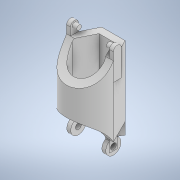
# Autodesk Inventor part: 검지_손가락_아래
Saved by Autodesk Inventor 2022 (Build 260153000, 153)
## iProperties
Created: 2023-11-18
Part Number: 검지_손가락_아래
Material: 일반
Document SubType Name: Modeling
Designer: USER
Density: 1 g/cm^3
Appearance: 기본값
Author: USER
Autodesk Inventor part; units mm, degrees
ref_plane "YZ Plane" through (0, 0, 0) normal (1, 0, 0) x (0, 1, 0)
ref_plane "XZ Plane" through (0, 0, 0) normal (0, 1, 0) x (-1, 0, 0)
ref_plane "XY Plane" through (0, 0, 0) normal (0, 0, 1) x (1, 0, 0)
sketch "스케치1" plane through (0, 0, 0) normal (0, 1, 0) x (-1, 0, 0)
  line L0 (0, 0) -> (0, -20)
  line L1 (0, -10) -> (-10, -10)
  line L2 (0, -20) -> (-5, -20)
  line L3 (-5, -20) -> (-10, -10)
  arc A0 (0, 0) -> (-10, -10) centre (0, -10) ccw
  line L4 (0, -20) -> (5, -20)
  line L5 (5, -20) -> (10, -10)
  arc A1 (10, -10) -> (0, 0) centre (0, -10) ccw
  dimension "d0" = 20
  dimension "d1" = 10
  dimension "d2" = 5
  constraints: 12 end point, 4 point on circle, 2 centre point, 2 horizontal, 2 symmetric about line, 1 coincident, 1 midpoint, 1 point on line, 1 vertical, 1 other
  measures "d0" distance of L0.start L0.end
  measures "d1" distance of L1.end L1.start
  measures "d2" distance of L0.end L2.end
extrude "돌출1" add sketch "스케치1" along normal blind 30
sketch "스케치7" plane through (0, 0, 0) normal (1, 0, 0) x (0, 1, 0)
  line L0 (30, -10) -> (30, 0) projected
  line L1 (30, 0) -> (21, 0)
  line L2 (0, 0) -> (30, 0) projected
  line L3 (21, 0) -> (25.4109, -9.3555) construction
  line L4 (25.4109, -9.3555) -> (35.2847, -12.2144) construction
  spline S0 degree 2 poles (21, 0) (25.4109, -9.3555) (35.2847, -12.2144) knots 1 1 1 2 2 2
  line L5 (35.2847, -12.2144) -> (35.2847, 0)
  line L6 (35.2847, 0) -> (21, 0)
  line L7 (15, 0) -> (15, 13.9402)
  line L8 (-5.2847, 0) -> (9, 0)
  line L9 (0, -10) -> (30, -10) projected
  line L10 (9, 0) -> (4.5891, -9.3555) construction
  line L11 (4.5891, -9.3555) -> (-5.2847, -12.2144) construction
  spline S1 degree 2 poles (9, 0) (4.5891, -9.3555) (-5.2847, -12.2144) knots 1 1 1 2 2 2
  line L12 (-5.2847, -12.2144) -> (-5.2847, 0)
  line L13 (-5.2847, 0) -> (9, 0)
  dimension "d22" = 9
  constraints: 14 end point, 4 symmetric about line, 2 vertical, 1 collinear, 1 midpoint, 1 point on line, 7 other
  measures "d22" distance of L0.end L1.end
extrude "돌출7" cut sketch "스케치7" along normal mid plane 30 contours S0 L1 L0 | L0 L6 L5 S0
shell "쉘2" thickness 3 removed faces 4 at (-1.6667, 0, -13.3333) at (0, 30, -16.6667) at (-4.9478, 27.2868, -8.1538) at (4.9478, 27.2869, -8.1538)
extrude "돌출8" cut sketch "스케치7" along normal mid plane 30 contours S1 L12 L8 L2
sketch "스케치8" plane through (0, 0, 0) normal (0, -1, 0) x (1, 0, 0)
  line L0 (10, -10) -> (5, -20) projected
  line L1 (6.6459, -10) -> (3.1459, -17) projected
  line L2 (10, -10) -> (6.6459, -10)
  line L3 (6.6459, -10) -> (8.3229, -10)
  line L4 (8.3229, -10) -> (8.3229, -13.3541)
  line L5 (8.3229, -13.3541) -> (6.6459, -13.3541)
  line L6 (6.6459, -13.3541) -> (6.6459, -10)
  line L7 (5, -20) -> (-5, -20) projected
  line L8 (0, -20) -> (0, -17)
  line L9 (-10, -10) -> (-6.6459, -10)
  line L10 (-8.3229, -10) -> (-8.3229, -13.3541)
  line L11 (-8.3229, -13.3541) -> (-6.6459, -13.3541)
  line L12 (-6.6459, -13.3541) -> (-6.6459, -10)
  point P0 (0, 0)
  constraints: 20 end point, 5 symmetric about line, 2 horizontal, 2 midpoint, 2 perpendicular, 1 point on line, 1 vertical
extrude "돌출9" add sketch "스케치8" along normal blind 5 contours L5 L6 L2 L4 | L9 L12 L11 L10
sketch "스케치9" plane through (0, 30, 0) normal (0, 1, 0) x (1, 0, 0)
  point P0 (0, 0)
sketch "스케치10" plane through (0, 30, 0) normal (0, 1, 0) x (1, 0, 0)
  line L0 (-5, 20) -> (-10, 10) projected
  line L1 (-6.6459, 10) -> (-8.3229, 10) projected
  line L2 (-10, 10) -> (-6.6459, 10)
  line L3 (-8.3229, 13.3541) -> (-8.3229, 10) projected
  line L4 (-8.3229, 10) -> (-8.3229, 13.3541)
  line L5 (-8.3229, 13.3541) -> (-10, 13.3541)
  line L6 (-10, 13.3541) -> (-10, 10)
  line L7 (5, 20) -> (-5, 20) projected
  line L8 (0, 20) -> (0, 17)
  line L9 (3.1459, 17) -> (-3.1459, 17) projected
  line L10 (10, 10) -> (6.6459, 10)
  line L11 (8.3229, 13.3541) -> (8.3229, 10)
  line L12 (8.3229, 13.3541) -> (10, 13.3541)
  line L13 (10, 13.3541) -> (10, 10)
  point P0 (0, 0)
  constraints: 18 end point, 5 symmetric about line, 2 collinear, 2 midpoint, 2 perpendicular
extrude "돌출10" add sketch "스케치10" along normal blind 5
sketch "스케치11" plane through (-8.3229, 30, -10) normal (1, 0, 0) x (0, 0, -1)
  line L0 (0, 5) -> (3.3541, 5) projected
  line L1 (0, -30) -> (0, 0) projected
  line L2 (3.3541, 5) -> (0, 5)
  line L3 (0, 5) -> (0, 0)
  line L4 (0, 0) -> (3.3541, 0)
  line L5 (3.3541, 0) -> (3.3541, 5)
  circle A0 centre (1.6771, 3.3229) radius 1.6771
  line L6 (3.3541, 0) -> (3.3541, 5) projected
  line L7 (0, 0) -> (0, 5) projected
  circle A1 centre (1.6771, 3.3229) radius 1
  point P0 (-10, -30)
  point P1 (0, 3.3229)
  point P2 (1.6771, 5)
  point P3 (3.3541, 3.3229)
  dimension "d32" = 2
  constraints: 8 end point, 3 tangent, 2 centre point, 2 parallel, 1 coincident, 1 horizontal, 1 perpendicular
  measures "d32" diameter of A1
sketch "스케치12" plane through (6.6459, 0, -13.3541) normal (-1, 0, 0) x (0, 0, 1)
  line L0 (0, 0) -> (0, -5) projected
  line L1 (3.3541, 0) -> (3.3541, -5) projected
  line L2 (0, -5) -> (3.3541, -5)
  line L3 (3.3541, -5) -> (3.3541, 0)
  line L4 (3.3541, 0) -> (0, 0)
  line L5 (0, 0) -> (0, -5)
  circle A0 centre (1.6771, -3.3229) radius 1.25
  circle A1 centre (1.6771, -3.3229) radius 3.25
  point P0 (13.3541, 0)
  point P1 (0, -0.5391)
  point P2 (3.3541, -0.5391)
  dimension "d33" = 2.5
  dimension "d57" = 6.5
  constraints: 8 end point, 2 centre point, 2 parallel, 1 coincident, 1 horizontal, 1 perpendicular
  measures "d33" diameter of A0
  measures "d57" diameter of A1
sketch "스케치13" plane through (0, 30, 0) normal (0, -1, 0) x (1, 0, 0)
  line L0 (10, -13.3541) -> (8.3229, -13.3541) projected
  line L1 (10, -10) -> (10, -13.3541) projected
  line L2 (10, -13.3541) -> (10, -10)
  line L3 (10, -10) -> (8.3229, -13.3541) projected
  line L4 (10, -10) -> (8.3229, -13.3541)
  line L5 (8.3229, -13.3541) -> (10, -13.3541)
  point P0 (0, 0)
  constraints: 6 end point, 2 collinear, 1 perpendicular
sketch "스케치14" plane through (0, 30, 0) normal (0, -1, 0) x (1, 0, 0)
  line L0 (-8.3229, -13.3541) -> (-10, -13.3541) projected
  line L1 (-10, -13.3541) -> (-10, -10) projected
  line L2 (-10, -13.3541) -> (-10, -10)
  line L3 (-8.3229, -13.3541) -> (-8.3229, -10) projected
  line L4 (-10, -10) -> (-8.3229, -13.3541)
  line L5 (-8.3229, -13.3541) -> (-10, -13.3541)
  point P0 (0, 0)
  constraints: 6 end point, 1 collinear, 1 perpendicular
extrude "돌출12" add sketch "스케치13" along normal blind 8
extrude "돌출13" add sketch "스케치14" along normal blind 8
sketch "스케치15" plane through (8.3229, 30, -13.3541) normal (-1, 0, 0) x (0, 0, 1)
  line L0 (3.3541, 0) -> (0, 0) projected
  line L1 (3.3541, 0) -> (3.3541, 5) projected
  line L2 (0, 5) -> (3.3541, 5) projected
  line L3 (0, 0) -> (0, 5) projected
  circle A0 centre (1.6771, 3.3229) radius 1 projected
  circle A1 centre (1.6771, 3.3229) radius 1.6771 projected
  point P0 (13.3541, -30)
extrude "돌출14" cut sketch "스케치11" along normal mid plane 100 contours L0 A0 L3 | L0 L5 A0
extrude "돌출15" add sketch "스케치11" along normal blind 2 contours A1
extrude "돌출16" add sketch "스케치15" along normal blind 2 contours A0
sketch "스케치16" plane through (0, 0, 0) normal (0, -1, 0) x (1, 0, 0)
  line L0 (5, -20) -> (-5, -20) projected
  line L1 (5, -20) -> (-5, -20)
  line L2 (-3.1459, -17) -> (3.1459, -17) projected
  line L3 (-5, -20) -> (-3.1459, -17)
  line L4 (3.1459, -17) -> (6.6459, -10) projected
  line L5 (-3.1459, -17) -> (3.1459, -17)
  line L6 (8.3229, -13.3541) -> (5, -20) projected
  line L7 (3.1459, -17) -> (5, -20)
  point P0 (0, 0)
  constraints: 8 end point, 1 collinear, 1 parallel
extrude "돌출17" add sketch "스케치16" along normal blind 5
ref_plane "작업 평면1" through (0, -5, 0) normal (0, 1, 0) x (-1, 0, 0)
extrude "돌출19" add sketch "스케치12" against normal blind 1.677 contours L0 L2 L1 A1 picked at (1.7841, -5.519)
extrude "돌출20" cut sketch "스케치12" against normal blind 2 contours A0
sketch "스케치18" plane through (-6.6459, 0, -10) normal (1, 0, 0) x (0, 0, -1)
  circle A0 centre (1.6771, -3.3229) radius 3.25 projected
  circle A1 centre (1.6771, -3.3229) radius 1.25 projected
  point P0 (-10, 0)
extrude "돌출21" add sketch "스케치18" against normal blind 1.677
extrude "돌출22" cut sketch "스케치12" along normal mid plane 50 contours A0
